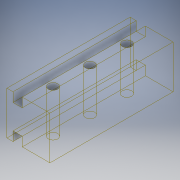
# Autodesk Inventor part: CLB_052_ScissorLiftPlug
Saved by Autodesk Inventor 2018.3 (Build 223284000, 284)
## iProperties
Created: 2020-02-14
Part Number: CLB_052_ScissorLiftPlug
Material: Nylon 6/6
Document SubType Name: Modeling
Designer: 22perngrac
Density: 1.13 g/cm^3
Appearance: Nylon 6
Mass: 31.4942 g
Surface Area: 93.6724 cm^2
Volume: 27.871 cm^3
Author: 22perngrac
Autodesk Inventor part; units mm, degrees
ref_plane "YZ Plane" through (0, 0, 0) normal (1, 0, 0) x (0, 1, 0)
ref_plane "XZ Plane" through (0, 0, 0) normal (0, 1, 0) x (-1, 0, 0)
ref_plane "XY Plane" through (0, 0, 0) normal (0, 0, 1) x (1, 0, 0)
sketch "Sketch1" plane through (0, 0, 0) normal (0, 0, 1) x (1, 0, 0)
  line L0 (0, 0) -> (22.225, 0)
  line L1 (22.225, 0) -> (22.225, 22.225)
  line L2 (22.225, 22.225) -> (0, 22.225)
  line L3 (0, 22.225) -> (0, 0)
  dimension "d0" = 22.225
  constraints: 8 end point, 2 parallel, 2 perpendicular, 1 horizontal
  measures "d0" distance of L1.end L2.end
extrude "Extrusion1" add sketch "Sketch1" along normal blind 63.5
sketch "Sketch2" plane through (0, 22.225, 0) normal (0, 1, 0) x (1, 0, 0)
  line L0 (0, 0) -> (0, -63.5) projected
  line L1 (22.225, -63.5) -> (0, -63.5) projected
  line L2 (22.225, 0) -> (0, 0) projected
  point P0 (11.1125, -12.7)
  point P1 (11.1125, -31.75)
  point P2 (11.1125, -50.8)
  point P3 (11.1125, 0)
  dimension "d26" = 12.7
  dimension "d28" = 19.05
  dimension "d29" = 19.05
  constraints: 3 vertical alignment, 1 midpoint
  measures "d26" distance from line of L2 point (11.113, -12.7)
  measures "d28" distance of point (11.113, -12.7) point (11.113, -31.75)
  measures "d29" distance of point (11.113, -31.75) point (11.113, -50.8)
hole "Hole1" at (11.1125, 22.225, 12.7) at (11.1125, 22.225, 31.75) at (11.1125, 22.225, 50.8) direction (0, -1, 0) diameter 4.8514 end through all
sketch "Sketch3" plane through (0, 0, 63.5) normal (0, 0, 1) x (1, 0, 0)
  line L0 (22.225, 22.225) -> (0, 22.225) projected
  line L1 (22.225, 0) -> (22.225, 22.225) projected
  line L2 (0, 22.225) -> (0, 0) projected
  line L3 (0, 0) -> (22.225, 0) projected
  point P0 (4.7625, 17.4625)
  point P1 (4.7625, 4.7625)
  dimension "d21" = 4.7625
  dimension "d22" = 4.7625
  dimension "d31" = 4.7625
  constraints: 1 vertical alignment
  measures "d21" distance from line of point (4.763, 17.463) L0
  measures "d22" distance from line of L2 point (4.763, 17.463)
  measures "d31" distance from line of point (4.763, 4.763) L3
hole "Hole2" [suppressed]
sketch "Sketch4" plane through (0, 0, 63.5) normal (0, 0, 1) x (1, 0, 0)
  line L0 (3.175, 27.2947) -> (7.9375, 27.2947)
  line L1 (7.9375, 27.2947) -> (7.9375, 17.4625)
  line L2 (7.9375, 17.4625) -> (3.175, 17.4625)
  line L3 (3.175, 17.4625) -> (3.175, 27.2947)
  line L4 (3.175, -4.5253) -> (7.9375, -4.5253)
  line L5 (7.9375, -4.5253) -> (7.9375, 4.7625)
  line L6 (7.9375, 4.7625) -> (3.175, 4.7625)
  line L7 (3.175, 4.7625) -> (3.175, -4.5253)
  line L8 (0, 0) -> (22.225, 0) projected
  line L9 (22.225, 22.225) -> (0, 22.225) projected
  line L10 (0, 22.225) -> (0, 0) projected
  dimension "d32" = 4.7625
  dimension "d33" = 4.7625
  dimension "d34" = 4.7625
  dimension "d35" = 7.9375
  dimension "d38" = 3.175
  constraints: 16 end point, 5 parallel, 2 horizontal, 2 perpendicular, 1 collinear
  measures "d32" distance of L0.start L0.end
  measures "d33" distance between parallel lines of L8 L6
  measures "d34" distance between parallel lines of L2 L9
  measures "d35" distance between parallel lines of L10 L5
  measures "d38" distance between parallel lines of L7 L10
extrude "Extrusion2" cut sketch "Sketch4" against normal through all
equation "\"d31\" = d21"
equation "\"d34\" = d33"
body "Solid1"
